Autodesk Inventor part; units mm, degrees
(part 3 of 3)
  point P86 (13.5104, 46.8405)
  point P87 (13.2211, 47.2236)
  point P88 (11.1615, 47.7468)
  point P89 (10.7263, 47.5553)
  point P90 (10.5426, 47.5964)
  point P91 (10.2298, 47.9606)
  point P92 (7.7191, 48.135)
  point P93 (7.5332, 48.1644)
  point P94 (7.1982, 48.5083)
  point P95 (5.0892, 48.7692)
  point P96 (4.6815, 48.5247)
  point P97 (4.4941, 48.5424)
  point P98 (4.1381, 48.8646)
  point P99 (2.0169, 48.9926)
  point P100 (1.6254, 48.7229)
  point P101 (1.4372, 48.7288)
  point P102 (1.0617, 49.028)
  point P103 (-1.0633, 49.0225)
  point P104 (-1.4372, 48.7288)
  point P105 (-1.6254, 48.7229)
  point P106 (-2.0189, 48.9979)
  point P107 (-2.8249, 50.9218)
  point P108 (-4.1394, 48.859)
  point P109 (-4.4941, 48.5424)
  point P110 (-4.6815, 48.5247)
  point P111 (-5.0915, 48.7745)
  point P112 (-6.0168, 50.6439)
  point P113 (-7.5332, 48.1644)
  point P114 (-7.7191, 48.135)
  point P115 (-8.144, 48.3585)
  point P116 (-9.1848, 50.1662)
  point P117 (-10.5426, 47.5964)
  point P118 (-10.7263, 47.5553)
  point P119 (-11.1644, 47.7517)
  point P120 (-12.3167, 49.4905)
  point P121 (-13.5104, 46.8405)
  point P122 (-13.6912, 46.788)
  point P123 (-14.1407, 46.9565)
  point P124 (-15.3999, 48.6194)
  point P125 (-16.1601, 46.2946)
  point P126 (-16.4249, 45.8997)
  point P127 (-16.602, 45.836)
  point P128 (-17.0612, 45.9759)
  point P129 (-18.4224, 47.5565)
  point P130 (-19.2745, 44.7778)
  point P131 (-19.4473, 44.7031)
  point P132 (-19.9144, 44.8139)
  point P133 (-21.3721, 46.3059)
  point P134 (-21.8349, 43.9042)
  point P135 (-22.0481, 43.4792)
  point P136 (-22.2159, 43.3938)
  point P137 (-24.2375, 44.8726)
  point P138 (-24.7347, 42.009)
  point P139 (-24.8967, 41.9132)
  point P140 (-25.3741, 41.9646)
  point P141 (-27.0072, 43.2622)
  point P142 (-27.1654, 40.8213)
  point P143 (-27.3237, 40.373)
  point P144 (-27.4794, 40.2672)
  point P145 (-27.959, 40.2885)
  point P146 (-29.6704, 41.481)
  point P147 (-29.6769, 39.0404)
  point P148 (-29.8048, 38.5777)
  point P149 (-29.9535, 38.4623)
  point P150 (-30.4336, 38.4535)
  point P151 (-32.0674, 37.0947)
  point P152 (-32.1683, 36.6301)
  point P153 (-32.3095, 36.5056)
  point P154 (-32.788, 36.4667)
  point P155 (-34.6354, 37.4352)
  point P156 (-34.4048, 34.5379)
  point P157 (-34.5379, 34.4048)
  point P158 (-35.0131, 34.3359)
  point P159 (-36.9176, 35.1866)
  point P160 (-36.5056, 32.3095)
  point P161 (-36.6301, 32.1683)
  point P162 (-37.1, 32.0697)
  point P163 (-39.0542, 32.7991)
  point P164 (-38.4623, 29.9535)
  point P165 (-38.5777, 29.8048)
  point P166 (-39.0404, 29.6769)
  point P167 (-41.0366, 30.2821)
  point P168 (-40.2851, 27.9545)
  point P169 (-40.2672, 27.4794)
  point P170 (-40.373, 27.3237)
  point P171 (-40.8268, 27.1669)
  point P172 (-42.857, 27.6457)
  point P173 (-41.9132, 24.8967)
  point P174 (-42.009, 24.7347)
  point P175 (-42.4521, 24.5498)
  point P176 (-43.471, 22.685)
  point P177 (-43.3938, 22.2159)
  point P178 (-43.4792, 22.0481)
  point P179 (-43.9098, 21.8358)
  point P180 (-45.984, 22.0563)
  point P181 (-44.7031, 19.4473)
  point P182 (-44.7778, 19.2745)
  point P183 (-45.1942, 19.0356)
  point P184 (-47.2782, 19.1254)
  point P185 (-45.836, 16.602)
  point P186 (-45.8997, 16.4249)
  point P187 (-46.3003, 16.1602)
  point P188 (-48.3858, 16.119)
  point P189 (-46.788, 13.6912)
  point P190 (-46.8405, 13.5104)
  point P191 (-47.2236, 13.2211)
  point P192 (-47.7468, 11.1615)
  point P193 (-47.5553, 10.7263)
  point P194 (-47.5964, 10.5426)
  point P195 (-47.9606, 10.2298)
  point P196 (-50.0245, 9.9276)
  point P197 (-48.135, 7.7191)
  point P198 (-48.1644, 7.5332)
  point P199 (-48.5083, 7.1982)
  constraints: 800 point on circle, 400 centre point, 600 other
extrude "Extrusion1" add sketch "Sketch1" along normal blind 7
sketch "Sketch10" plane through (0, 0, 7) normal (0, 0, 1) x (1, 0, 0)
  arc A0 (6.577, -1.5182) -> (6.6574, -1.1143) centre (0, 0) ccw
  arc A1 (7.0958, -0.7827) -> (6.6574, -1.1143) centre (7.0519, -1.1803) ccw
  line L0 (7.0958, -0.7827) -> (7.489, -0.8261)
  spline S0 degree 3 poles (7.489, -0.8261) (7.5332, -0.828) (7.6661, -0.828) (7.8888, -0.7776) knots 0 0 0 0 1 1 1 1
  line L1 (7.489, -0.8261) -> (7.5332, -0.828) construction
  line L2 (7.5332, -0.828) -> (7.6661, -0.828) construction
  line L3 (7.6661, -0.828) -> (7.8888, -0.7776) construction
  spline S1 degree 3 poles (7.8888, -0.7776) (8.1533, -0.7172) (8.5333, -0.5858) (8.996, -0.3043) knots 0 0 0 0 1 1 1 1
  line L4 (7.8888, -0.7776) -> (8.1533, -0.7172) construction
  line L5 (8.1533, -0.7172) -> (8.5333, -0.5858) construction
  line L6 (8.5333, -0.5858) -> (8.996, -0.3043) construction
  arc A2 (8.996, -0.3043) -> (8.996, 0.3043) centre (0, 0) ccw
  spline S2 degree 3 poles (8.996, 0.3043) (8.5333, 0.5858) (8.1533, 0.7172) (7.8888, 0.7776) knots 0 0 0 0 1 1 1 1
  line L7 (8.996, 0.3043) -> (8.5333, 0.5858) construction
  line L8 (8.5333, 0.5858) -> (8.1533, 0.7172) construction
  line L9 (8.1533, 0.7172) -> (7.8888, 0.7776) construction
  spline S3 degree 3 poles (7.8888, 0.7776) (7.6661, 0.828) (7.5332, 0.828) (7.489, 0.8261) knots 0 0 0 0 1 1 1 1
  line L10 (7.8888, 0.7776) -> (7.6661, 0.828) construction
  line L11 (7.6661, 0.828) -> (7.5332, 0.828) construction
  line L12 (7.5332, 0.828) -> (7.489, 0.8261) construction
  line L13 (7.489, 0.8261) -> (7.0958, 0.7827)
  arc A3 (6.6574, 1.1143) -> (7.0958, 0.7827) centre (7.0519, 1.1803) ccw
  arc A4 (6.6574, 1.1143) -> (6.577, 1.5182) centre (0, 0) ccw
  arc A5 (6.8552, 1.9923) -> (6.577, 1.5182) centre (6.9668, 1.6082) ccw
  line L14 (6.8552, 1.9923) -> (7.2351, 2.1027)
  spline S4 degree 3 poles (7.2351, 2.1027) (7.2766, 2.1178) (7.3994, 2.1687) (7.5858, 2.3005) knots 0 0 0 0 1 1 1 1
  line L15 (7.2351, 2.1027) -> (7.2766, 2.1178) construction
  line L16 (7.2766, 2.1178) -> (7.3994, 2.1687) construction
  line L17 (7.3994, 2.1687) -> (7.5858, 2.3005) construction
  spline S5 degree 3 poles (7.5858, 2.3005) (7.8072, 2.4576) (8.1079, 2.7244) (8.4277, 3.1615) knots 0 0 0 0 1 1 1 1
  line L18 (7.5858, 2.3005) -> (7.8072, 2.4576) construction
  line L19 (7.8072, 2.4576) -> (8.1079, 2.7244) construction
  line L20 (8.1079, 2.7244) -> (8.4277, 3.1615) construction
  arc A6 (8.4277, 3.1615) -> (8.1948, 3.7238) centre (0, 0) ccw
  spline S6 degree 3 poles (8.1948, 3.7238) (7.6596, 3.8067) (7.2583, 3.7827) (6.9907, 3.7373) knots 0 0 0 0 1 1 1 1
  line L21 (8.1948, 3.7238) -> (7.6596, 3.8067) construction
  line L22 (7.6596, 3.8067) -> (7.2583, 3.7827) construction
  line L23 (7.2583, 3.7827) -> (6.9907, 3.7373) construction
  spline S7 degree 3 poles (6.9907, 3.7373) (6.7657, 3.6986) (6.6429, 3.6478) (6.6028, 3.6291) knots 0 0 0 0 1 1 1 1
  line L24 (6.9907, 3.7373) -> (6.7657, 3.6986) construction
  line L25 (6.7657, 3.6986) -> (6.6429, 3.6478) construction
  line L26 (6.6429, 3.6478) -> (6.6028, 3.6291) construction
  line L27 (6.6028, 3.6291) -> (6.2561, 3.4386)
  arc A7 (5.7242, 3.5771) -> (6.2561, 3.4386) centre (6.0634, 3.7891) ccw
  arc A8 (5.7242, 3.5771) -> (5.4954, 3.9196) centre (0, 0) ccw
  arc A9 (5.5709, 4.464) -> (5.4954, 3.9196) centre (5.8211, 4.1518) ccw
  line L28 (5.5709, 4.464) -> (5.8797, 4.7114)
  spline S8 degree 3 poles (5.8797, 4.7114) (5.9123, 4.7413) (6.0062, 4.8353) (6.128, 5.0284) knots 0 0 0 0 1 1 1 1
  line L29 (5.8797, 4.7114) -> (5.9123, 4.7413) construction
  line L30 (5.9123, 4.7413) -> (6.0062, 4.8353) construction
  line L31 (6.0062, 4.8353) -> (6.128, 5.0284) construction
  spline S9 degree 3 poles (6.128, 5.0284) (6.2724, 5.2582) (6.4481, 5.6197) (6.5763, 6.146) knots 0 0 0 0 1 1 1 1
  line L32 (6.128, 5.0284) -> (6.2724, 5.2582) construction
  line L33 (6.2724, 5.2582) -> (6.4481, 5.6197) construction
  line L34 (6.4481, 5.6197) -> (6.5763, 6.146) construction
  arc A10 (6.5763, 6.146) -> (6.146, 6.5763) centre (0, 0) ccw
  spline S10 degree 3 poles (6.146, 6.5763) (5.6197, 6.4481) (5.2582, 6.2724) (5.0284, 6.128) knots 0 0 0 0 1 1 1 1
  line L35 (6.146, 6.5763) -> (5.6197, 6.4481) construction
  line L36 (5.6197, 6.4481) -> (5.2582, 6.2724) construction
  line L37 (5.2582, 6.2724) -> (5.0284, 6.128) construction
  spline S11 degree 3 poles (5.0284, 6.128) (4.8353, 6.0062) (4.7413, 5.9123) (4.7114, 5.8797) knots 0 0 0 0 1 1 1 1
  line L38 (5.0284, 6.128) -> (4.8353, 6.0062) construction
  line L39 (4.8353, 6.0062) -> (4.7413, 5.9123) construction
  line L40 (4.7413, 5.9123) -> (4.7114, 5.8797) construction
  line L41 (4.7114, 5.8797) -> (4.464, 5.5709)
  arc A11 (3.9196, 5.4954) -> (4.464, 5.5709) centre (4.1518, 5.8211) ccw
  arc A12 (3.9196, 5.4954) -> (3.5771, 5.7242) centre (0, 0) ccw
  arc A13 (3.4386, 6.2561) -> (3.5771, 5.7242) centre (3.7891, 6.0634) ccw
  line L42 (3.4386, 6.2561) -> (3.6291, 6.6028)
  spline S12 degree 3 poles (3.6291, 6.6028) (3.6478, 6.6429) (3.6986, 6.7657) (3.7373, 6.9907) knots 0 0 0 0 1 1 1 1
  line L43 (3.6291, 6.6028) -> (3.6478, 6.6429) construction
  line L44 (3.6478, 6.6429) -> (3.6986, 6.7657) construction
  line L45 (3.6986, 6.7657) -> (3.7373, 6.9907) construction
  spline S13 degree 3 poles (3.7373, 6.9907) (3.7827, 7.2583) (3.8067, 7.6596) (3.7238, 8.1948) knots 0 0 0 0 1 1 1 1
  line L46 (3.7373, 6.9907) -> (3.7827, 7.2583) construction
  line L47 (3.7827, 7.2583) -> (3.8067, 7.6596) construction
  line L48 (3.8067, 7.6596) -> (3.7238, 8.1948) construction
  arc A14 (3.7238, 8.1948) -> (3.1615, 8.4277) centre (0, 0) ccw
  spline S14 degree 3 poles (3.1615, 8.4277) (2.7244, 8.1079) (2.4576, 7.8072) (2.3005, 7.5858) knots 0 0 0 0 1 1 1 1
  line L49 (3.1615, 8.4277) -> (2.7244, 8.1079) construction
  line L50 (2.7244, 8.1079) -> (2.4576, 7.8072) construction
  line L51 (2.4576, 7.8072) -> (2.3005, 7.5858) construction
  spline S15 degree 3 poles (2.3005, 7.5858) (2.1687, 7.3994) (2.1178, 7.2766) (2.1027, 7.2351) knots 0 0 0 0 1 1 1 1
  line L52 (2.3005, 7.5858) -> (2.1687, 7.3994) construction
  line L53 (2.1687, 7.3994) -> (2.1178, 7.2766) construction
  line L54 (2.1178, 7.2766) -> (2.1027, 7.2351) construction
  line L55 (2.1027, 7.2351) -> (1.9923, 6.8552)
  arc A15 (1.5182, 6.577) -> (1.9923, 6.8552) centre (1.6082, 6.9668) ccw
  arc A16 (1.5182, 6.577) -> (1.1143, 6.6574) centre (0, 0) ccw
  arc A17 (0.7827, 7.0958) -> (1.1143, 6.6574) centre (1.1803, 7.0519) ccw
  line L56 (0.7827, 7.0958) -> (0.8261, 7.489)
  spline S16 degree 3 poles (0.8261, 7.489) (0.828, 7.5332) (0.828, 7.6661) (0.7776, 7.8888) knots 0 0 0 0 1 1 1 1
  line L57 (0.8261, 7.489) -> (0.828, 7.5332) construction
  line L58 (0.828, 7.5332) -> (0.828, 7.6661) construction
  line L59 (0.828, 7.6661) -> (0.7776, 7.8888) construction
  spline S17 degree 3 poles (0.7776, 7.8888) (0.7172, 8.1533) (0.5858, 8.5333) (0.3043, 8.996) knots 0 0 0 0 1 1 1 1
  line L60 (0.7776, 7.8888) -> (0.7172, 8.1533) construction
  line L61 (0.7172, 8.1533) -> (0.5858, 8.5333) construction
  line L62 (0.5858, 8.5333) -> (0.3043, 8.996) construction
  arc A18 (0.3043, 8.996) -> (-0.3043, 8.996) centre (0, 0) ccw
  spline S18 degree 3 poles (-0.3043, 8.996) (-0.5858, 8.5333) (-0.7172, 8.1533) (-0.7776, 7.8888) knots 0 0 0 0 1 1 1 1
  line L63 (-0.3043, 8.996) -> (-0.5858, 8.5333) construction
  line L64 (-0.5858, 8.5333) -> (-0.7172, 8.1533) construction
  line L65 (-0.7172, 8.1533) -> (-0.7776, 7.8888) construction
  spline S19 degree 3 poles (-0.7776, 7.8888) (-0.828, 7.6661) (-0.828, 7.5332) (-0.8261, 7.489) knots 0 0 0 0 1 1 1 1
  line L66 (-0.7776, 7.8888) -> (-0.828, 7.6661) construction
  line L67 (-0.828, 7.6661) -> (-0.828, 7.5332) construction
  line L68 (-0.828, 7.5332) -> (-0.8261, 7.489) construction
  line L69 (-0.8261, 7.489) -> (-0.7827, 7.0958)
  arc A19 (-1.1143, 6.6574) -> (-0.7827, 7.0958) centre (-1.1803, 7.0519) ccw
  arc A20 (-1.1143, 6.6574) -> (-1.5182, 6.577) centre (0, 0) ccw
  arc A21 (-1.9923, 6.8552) -> (-1.5182, 6.577) centre (-1.6082, 6.9668) ccw
  line L70 (-1.9923, 6.8552) -> (-2.1027, 7.2351)
  spline S20 degree 3 poles (-2.1027, 7.2351) (-2.1178, 7.2766) (-2.1687, 7.3994) (-2.3005, 7.5858) knots 0 0 0 0 1 1 1 1
  line L71 (-2.1027, 7.2351) -> (-2.1178, 7.2766) construction
  line L72 (-2.1178, 7.2766) -> (-2.1687, 7.3994) construction
  line L73 (-2.1687, 7.3994) -> (-2.3005, 7.5858) construction
  spline S21 degree 3 poles (-2.3005, 7.5858) (-2.4576, 7.8072) (-2.7244, 8.1079) (-3.1615, 8.4277) knots 0 0 0 0 1 1 1 1
  line L74 (-2.3005, 7.5858) -> (-2.4576, 7.8072) construction
  line L75 (-2.4576, 7.8072) -> (-2.7244, 8.1079) construction
  line L76 (-2.7244, 8.1079) -> (-3.1615, 8.4277) construction
  arc A22 (-3.1615, 8.4277) -> (-3.7238, 8.1948) centre (0, 0) ccw
  spline S22 degree 3 poles (-3.7238, 8.1948) (-3.8067, 7.6596) (-3.7827, 7.2583) (-3.7373, 6.9907) knots 0 0 0 0 1 1 1 1
  line L77 (-3.7238, 8.1948) -> (-3.8067, 7.6596) construction
  line L78 (-3.8067, 7.6596) -> (-3.7827, 7.2583) construction
  line L79 (-3.7827, 7.2583) -> (-3.7373, 6.9907) construction
  spline S23 degree 3 poles (-3.7373, 6.9907) (-3.6986, 6.7657) (-3.6478, 6.6429) (-3.6291, 6.6028) knots 0 0 0 0 1 1 1 1
  line L80 (-3.7373, 6.9907) -> (-3.6986, 6.7657) construction
  line L81 (-3.6986, 6.7657) -> (-3.6478, 6.6429) construction
  line L82 (-3.6478, 6.6429) -> (-3.6291, 6.6028) construction
  line L83 (-3.6291, 6.6028) -> (-3.4386, 6.2561)
  arc A23 (-3.5771, 5.7242) -> (-3.4386, 6.2561) centre (-3.7891, 6.0634) ccw
  arc A24 (-3.5771, 5.7242) -> (-3.9196, 5.4954) centre (0, 0) ccw
  arc A25 (-4.464, 5.5709) -> (-3.9196, 5.4954) centre (-4.1518, 5.8211) ccw
  line L84 (-4.464, 5.5709) -> (-4.7114, 5.8797)
  spline S24 degree 3 poles (-4.7114, 5.8797) (-4.7413, 5.9123) (-4.8353, 6.0062) (-5.0284, 6.128) knots 0 0 0 0 1 1 1 1
  line L85 (-4.7114, 5.8797) -> (-4.7413, 5.9123) construction
  line L86 (-4.7413, 5.9123) -> (-4.8353, 6.0062) construction
  line L87 (-4.8353, 6.0062) -> (-5.0284, 6.128) construction
  spline S25 degree 3 poles (-5.0284, 6.128) (-5.2582, 6.2724) (-5.6197, 6.4481) (-6.146, 6.5763) knots 0 0 0 0 1 1 1 1
  line L88 (-5.0284, 6.128) -> (-5.2582, 6.2724) construction
  line L89 (-5.2582, 6.2724) -> (-5.6197, 6.4481) construction
  line L90 (-5.6197, 6.4481) -> (-6.146, 6.5763) construction
  arc A26 (-6.146, 6.5763) -> (-6.5763, 6.146) centre (0, 0) ccw
  spline S26 degree 3 poles (-6.5763, 6.146) (-6.4481, 5.6197) (-6.2724, 5.2582) (-6.128, 5.0284) knots 0 0 0 0 1 1 1 1
  line L91 (-6.5763, 6.146) -> (-6.4481, 5.6197) construction
  line L92 (-6.4481, 5.6197) -> (-6.2724, 5.2582) construction
  line L93 (-6.2724, 5.2582) -> (-6.128, 5.0284) construction
  spline S27 degree 3 poles (-6.128, 5.0284) (-6.0062, 4.8353) (-5.9123, 4.7413) (-5.8797, 4.7114) knots 0 0 0 0 1 1 1 1
  line L94 (-6.128, 5.0284) -> (-6.0062, 4.8353) construction
  line L95 (-6.0062, 4.8353) -> (-5.9123, 4.7413) construction
  line L96 (-5.9123, 4.7413) -> (-5.8797, 4.7114) construction
  line L97 (-5.8797, 4.7114) -> (-5.5709, 4.464)
  arc A27 (-5.4954, 3.9196) -> (-5.5709, 4.464) centre (-5.8211, 4.1518) ccw
  arc A28 (-5.4954, 3.9196) -> (-5.7242, 3.5771) centre (0, 0) ccw
  arc A29 (-6.2561, 3.4386) -> (-5.7242, 3.5771) centre (-6.0634, 3.7891) ccw
  line L98 (-6.2561, 3.4386) -> (-6.6028, 3.6291)
  spline S28 degree 3 poles (-6.6028, 3.6291) (-6.6429, 3.6478) (-6.7657, 3.6986) (-6.9907, 3.7373) knots 0 0 0 0 1 1 1 1
  line L99 (-6.6028, 3.6291) -> (-6.6429, 3.6478) construction
  line L100 (-6.6429, 3.6478) -> (-6.7657, 3.6986) construction
  line L101 (-6.7657, 3.6986) -> (-6.9907, 3.7373) construction
  spline S29 degree 3 poles (-6.9907, 3.7373) (-7.2583, 3.7827) (-7.6596, 3.8067) (-8.1948, 3.7238) knots 0 0 0 0 1 1 1 1
  line L102 (-6.9907, 3.7373) -> (-7.2583, 3.7827) construction
  line L103 (-7.2583, 3.7827) -> (-7.6596, 3.8067) construction
  line L104 (-7.6596, 3.8067) -> (-8.1948, 3.7238) construction
  arc A30 (-8.1948, 3.7238) -> (-8.4277, 3.1615) centre (0, 0) ccw
  spline S30 degree 3 poles (-8.4277, 3.1615) (-8.1079, 2.7244) (-7.8072, 2.4576) (-7.5858, 2.3005) knots 0 0 0 0 1 1 1 1
  line L105 (-8.4277, 3.1615) -> (-8.1079, 2.7244) construction
  line L106 (-8.1079, 2.7244) -> (-7.8072, 2.4576) construction
  line L107 (-7.8072, 2.4576) -> (-7.5858, 2.3005) construction
  spline S31 degree 3 poles (-7.5858, 2.3005) (-7.3994, 2.1687) (-7.2766, 2.1178) (-7.2351, 2.1027) knots 0 0 0 0 1 1 1 1
  line L108 (-7.5858, 2.3005) -> (-7.3994, 2.1687) construction
  line L109 (-7.3994, 2.1687) -> (-7.2766, 2.1178) construction
  line L110 (-7.2766, 2.1178) -> (-7.2351, 2.1027) construction
  line L111 (-7.2351, 2.1027) -> (-6.8552, 1.9923)
  arc A31 (-6.577, 1.5182) -> (-6.8552, 1.9923) centre (-6.9668, 1.6082) ccw
  arc A32 (-6.577, 1.5182) -> (-6.6574, 1.1143) centre (0, 0) ccw
  arc A33 (-7.0958, 0.7827) -> (-6.6574, 1.1143) centre (-7.0519, 1.1803) ccw
  line L112 (-7.0958, 0.7827) -> (-7.489, 0.8261)
  spline S32 degree 3 poles (-7.489, 0.8261) (-7.5332, 0.828) (-7.6661, 0.828) (-7.8888, 0.7776) knots 0 0 0 0 1 1 1 1
  line L113 (-7.489, 0.8261) -> (-7.5332, 0.828) construction
  line L114 (-7.5332, 0.828) -> (-7.6661, 0.828) construction
  line L115 (-7.6661, 0.828) -> (-7.8888, 0.7776) construction
  spline S33 degree 3 poles (-7.8888, 0.7776) (-8.1533, 0.7172) (-8.5333, 0.5858) (-8.996, 0.3043) knots 0 0 0 0 1 1 1 1
  line L116 (-7.8888, 0.7776) -> (-8.1533, 0.7172) construction
  line L117 (-8.1533, 0.7172) -> (-8.5333, 0.5858) construction
  line L118 (-8.5333, 0.5858) -> (-8.996, 0.3043) construction
  arc A34 (-8.996, 0.3043) -> (-8.996, -0.3043) centre (0, 0) ccw
  spline S34 degree 3 poles (-8.996, -0.3043) (-8.5333, -0.5858) (-8.1533, -0.7172) (-7.8888, -0.7776) knots 0 0 0 0 1 1 1 1
  line L119 (-8.996, -0.3043) -> (-8.5333, -0.5858) construction
  line L120 (-8.5333, -0.5858) -> (-8.1533, -0.7172) construction
  line L121 (-8.1533, -0.7172) -> (-7.8888, -0.7776) construction
  spline S35 degree 3 poles (-7.8888, -0.7776) (-7.6661, -0.828) (-7.5332, -0.828) (-7.489, -0.8261) knots 0 0 0 0 1 1 1 1
  line L122 (-7.8888, -0.7776) -> (-7.6661, -0.828) construction
  line L123 (-7.6661, -0.828) -> (-7.5332, -0.828) construction
  line L124 (-7.5332, -0.828) -> (-7.489, -0.8261) construction
  line L125 (-7.489, -0.8261) -> (-7.0958, -0.7827)
  arc A35 (-6.6574, -1.1143) -> (-7.0958, -0.7827) centre (-7.0519, -1.1803) ccw
  arc A36 (-6.6574, -1.1143) -> (-6.577, -1.5182) centre (0, 0) ccw
  arc A37 (-6.8552, -1.9923) -> (-6.577, -1.5182) centre (-6.9668, -1.6082) ccw
  line L126 (-6.8552, -1.9923) -> (-7.2351, -2.1027)
  spline S36 degree 3 poles (-7.2351, -2.1027) (-7.2766, -2.1178) (-7.3994, -2.1687) (-7.5858, -2.3005) knots 0 0 0 0 1 1 1 1
  line L127 (-7.2351, -2.1027) -> (-7.2766, -2.1178) construction
  line L128 (-7.2766, -2.1178) -> (-7.3994, -2.1687) construction
  line L129 (-7.3994, -2.1687) -> (-7.5858, -2.3005) construction
  spline S37 degree 3 poles (-7.5858, -2.3005) (-7.8072, -2.4576) (-8.1079, -2.7244) (-8.4277, -3.1615) knots 0 0 0 0 1 1 1 1
  line L130 (-7.5858, -2.3005) -> (-7.8072, -2.4576) construction
  line L131 (-7.8072, -2.4576) -> (-8.1079, -2.7244) construction
  line L132 (-8.1079, -2.7244) -> (-8.4277, -3.1615) construction
  arc A38 (-8.4277, -3.1615) -> (-8.1948, -3.7238) centre (0, 0) ccw
  spline S38 degree 3 poles (-8.1948, -3.7238) (-7.6596, -3.8067) (-7.2583, -3.7827) (-6.9907, -3.7373) knots 0 0 0 0 1 1 1 1
  line L133 (-8.1948, -3.7238) -> (-7.6596, -3.8067) construction
  line L134 (-7.6596, -3.8067) -> (-7.2583, -3.7827) construction
  line L135 (-7.2583, -3.7827) -> (-6.9907, -3.7373) construction
  spline S39 degree 3 poles (-6.9907, -3.7373) (-6.7657, -3.6986) (-6.6429, -3.6478) (-6.6028, -3.6291) knots 0 0 0 0 1 1 1 1
  line L136 (-6.9907, -3.7373) -> (-6.7657, -3.6986) construction
  line L137 (-6.7657, -3.6986) -> (-6.6429, -3.6478) construction
  line L138 (-6.6429, -3.6478) -> (-6.6028, -3.6291) construction
  line L139 (-6.6028, -3.6291) -> (-6.2561, -3.4386)
  arc A39 (-5.7242, -3.5771) -> (-6.2561, -3.4386) centre (-6.0634, -3.7891) ccw
  arc A40 (-5.7242, -3.5771) -> (-5.4954, -3.9196) centre (0, 0) ccw
  arc A41 (-5.5709, -4.464) -> (-5.4954, -3.9196) centre (-5.8211, -4.1518) ccw
  line L140 (-5.5709, -4.464) -> (-5.8797, -4.7114)
  spline S40 degree 3 poles (-5.8797, -4.7114) (-5.9123, -4.7413) (-6.0062, -4.8353) (-6.128, -5.0284) knots 0 0 0 0 1 1 1 1
  line L141 (-5.8797, -4.7114) -> (-5.9123, -4.7413) construction
  line L142 (-5.9123, -4.7413) -> (-6.0062, -4.8353) construction
  line L143 (-6.0062, -4.8353) -> (-6.128, -5.0284) construction
  spline S41 degree 3 poles (-6.128, -5.0284) (-6.2724, -5.2582) (-6.4481, -5.6197) (-6.5763, -6.146) knots 0 0 0 0 1 1 1 1
  line L144 (-6.128, -5.0284) -> (-6.2724, -5.2582) construction
  line L145 (-6.2724, -5.2582) -> (-6.4481, -5.6197) construction
  line L146 (-6.4481, -5.6197) -> (-6.5763, -6.146) construction
  arc A42 (-6.5763, -6.146) -> (-6.146, -6.5763) centre (0, 0) ccw
  spline S42 degree 3 poles (-6.146, -6.5763) (-5.6197, -6.4481) (-5.2582, -6.2724) (-5.0284, -6.128) knots 0 0 0 0 1 1 1 1
  line L147 (-6.146, -6.5763) -> (-5.6197, -6.4481) construction
  line L148 (-5.6197, -6.4481) -> (-5.2582, -6.2724) construction
  line L149 (-5.2582, -6.2724) -> (-5.0284, -6.128) construction
  spline S43 degree 3 poles (-5.0284, -6.128) (-4.8353, -6.0062) (-4.7413, -5.9123) (-4.7114, -5.8797) knots 0 0 0 0 1 1 1 1
  line L150 (-5.0284, -6.128) -> (-4.8353, -6.0062) construction
  line L151 (-4.8353, -6.0062) -> (-4.7413, -5.9123) construction
  line L152 (-4.7413, -5.9123) -> (-4.7114, -5.8797) construction
  line L153 (-4.7114, -5.8797) -> (-4.464, -5.5709)
  arc A43 (-3.9196, -5.4954) -> (-4.464, -5.5709) centre (-4.1518, -5.8211) ccw
  arc A44 (-3.9196, -5.4954) -> (-3.5771, -5.7242) centre (0, 0) ccw
  arc A45 (-3.4386, -6.2561) -> (-3.5771, -5.7242) centre (-3.7891, -6.0634) ccw
  line L154 (-3.4386, -6.2561) -> (-3.6291, -6.6028)
  spline S44 degree 3 poles (-3.6291, -6.6028) (-3.6478, -6.6429) (-3.6986, -6.7657) (-3.7373, -6.9907) knots 0 0 0 0 1 1 1 1
  line L155 (-3.6291, -6.6028) -> (-3.6478, -6.6429) construction
  line L156 (-3.6478, -6.6429) -> (-3.6986, -6.7657) construction
  line L157 (-3.6986, -6.7657) -> (-3.7373, -6.9907) construction
  spline S45 degree 3 poles (-3.7373, -6.9907) (-3.7827, -7.2583) (-3.8067, -7.6596) (-3.7238, -8.1948) knots 0 0 0 0 1 1 1 1
  line L158 (-3.7373, -6.9907) -> (-3.7827, -7.2583) construction
  line L159 (-3.7827, -7.2583) -> (-3.8067, -7.6596) construction
  line L160 (-3.8067, -7.6596) -> (-3.7238, -8.1948) construction
  arc A46 (-3.7238, -8.1948) -> (-3.1615, -8.4277) centre (0, 0) ccw
  spline S46 degree 3 poles (-3.1615, -8.4277) (-2.7244, -8.1079) (-2.4576, -7.8072) (-2.3005, -7.5858) knots 0 0 0 0 1 1 1 1
  line L161 (-3.1615, -8.4277) -> (-2.7244, -8.1079) construction
  line L162 (-2.7244, -8.1079) -> (-2.4576, -7.8072) construction
  line L163 (-2.4576, -7.8072) -> (-2.3005, -7.5858) construction
  spline S47 degree 3 poles (-2.3005, -7.5858) (-2.1687, -7.3994) (-2.1178, -7.2766) (-2.1027, -7.2351) knots 0 0 0 0 1 1 1 1
  line L164 (-2.3005, -7.5858) -> (-2.1687, -7.3994) construction
  line L165 (-2.1687, -7.3994) -> (-2.1178, -7.2766) construction
  line L166 (-2.1178, -7.2766) -> (-2.1027, -7.2351) construction
  line L167 (-2.1027, -7.2351) -> (-1.9923, -6.8552)
  arc A47 (-1.5182, -6.577) -> (-1.9923, -6.8552) centre (-1.6082, -6.9668) ccw
  arc A48 (-1.5182, -6.577) -> (-1.1143, -6.6574) centre (0, 0) ccw
  arc A49 (-0.7827, -7.0958) -> (-1.1143, -6.6574) centre (-1.1803, -7.0519) ccw
  line L168 (-0.7827, -7.0958) -> (-0.8261, -7.489)
  spline S48 degree 3 poles (-0.8261, -7.489) (-0.828, -7.5332) (-0.828, -7.6661) (-0.7776, -7.8888) knots 0 0 0 0 1 1 1 1
  line L169 (-0.8261, -7.489) -> (-0.828, -7.5332) construction
  line L170 (-0.828, -7.5332) -> (-0.828, -7.6661) construction
  line L171 (-0.828, -7.6661) -> (-0.7776, -7.8888) construction
  spline S49 degree 3 poles (-0.7776, -7.8888) (-0.7172, -8.1533) (-0.5858, -8.5333) (-0.3043, -8.996) knots 0 0 0 0 1 1 1 1
  line L172 (-0.7776, -7.8888) -> (-0.7172, -8.1533) construction
  line L173 (-0.7172, -8.1533) -> (-0.5858, -8.5333) construction
  line L174 (-0.5858, -8.5333) -> (-0.3043, -8.996) construction
  arc A50 (-0.3043, -8.996) -> (0.3043, -8.996) centre (0, 0) ccw
  spline S50 degree 3 poles (0.3043, -8.996) (0.5858, -8.5333) (0.7172, -8.1533) (0.7776, -7.8888) knots 0 0 0 0 1 1 1 1
  line L175 (0.3043, -8.996) -> (0.5858, -8.5333) construction
  line L176 (0.5858, -8.5333) -> (0.7172, -8.1533) construction
  line L177 (0.7172, -8.1533) -> (0.7776, -7.8888) construction
  spline S51 degree 3 poles (0.7776, -7.8888) (0.828, -7.6661) (0.828, -7.5332) (0.8261, -7.489) knots 0 0 0 0 1 1 1 1
  line L178 (0.7776, -7.8888) -> (0.828, -7.6661) construction
  line L179 (0.828, -7.6661) -> (0.828, -7.5332) construction
  line L180 (0.828, -7.5332) -> (0.8261, -7.489) construction
  line L181 (0.8261, -7.489) -> (0.7827, -7.0958)
  arc A51 (1.1143, -6.6574) -> (0.7827, -7.0958) centre (1.1803, -7.0519) ccw
  arc A52 (1.1143, -6.6574) -> (1.5182, -6.577) centre (0, 0) ccw
  arc A53 (1.9923, -6.8552) -> (1.5182, -6.577) centre (1.6082, -6.9668) ccw
  line L182 (1.9923, -6.8552) -> (2.1027, -7.2351)
  spline S52 degree 3 poles (2.1027, -7.2351) (2.1178, -7.2766) (2.1687, -7.3994) (2.3005, -7.5858) knots 0 0 0 0 1 1 1 1
  line L183 (2.1027, -7.2351) -> (2.1178, -7.2766) construction
  line L184 (2.1178, -7.2766) -> (2.1687, -7.3994) construction
  line L185 (2.1687, -7.3994) -> (2.3005, -7.5858) construction
  spline S53 degree 3 poles (2.3005, -7.5858) (2.4576, -7.8072) (2.7244, -8.1079) (3.1615, -8.4277) knots 0 0 0 0 1 1 1 1
  line L186 (2.3005, -7.5858) -> (2.4576, -7.8072) construction
  line L187 (2.4576, -7.8072) -> (2.7244, -8.1079) construction
  line L188 (2.7244, -8.1079) -> (3.1615, -8.4277) construction
  arc A54 (3.1615, -8.4277) -> (3.7238, -8.1948) centre (0, 0) ccw
  spline S54 degree 3 poles (3.7238, -8.1948) (3.8067, -7.6596) (3.7827, -7.2583) (3.7373, -6.9907) knots 0 0 0 0 1 1 1 1
  line L189 (3.7238, -8.1948) -> (3.8067, -7.6596) construction
  line L190 (3.8067, -7.6596) -> (3.7827, -7.2583) construction
  line L191 (3.7827, -7.2583) -> (3.7373, -6.9907) construction
  spline S55 degree 3 poles (3.7373, -6.9907) (3.6986, -6.7657) (3.6478, -6.6429) (3.6291, -6.6028) knots 0 0 0 0 1 1 1 1
  line L192 (3.7373, -6.9907) -> (3.6986, -6.7657) construction
  line L193 (3.6986, -6.7657) -> (3.6478, -6.6429) construction
  line L194 (3.6478, -6.6429) -> (3.6291, -6.6028) construction
  line L195 (3.6291, -6.6028) -> (3.4386, -6.2561)
  arc A55 (3.5771, -5.7242) -> (3.4386, -6.2561) centre (3.7891, -6.0634) ccw
  arc A56 (3.5771, -5.7242) -> (3.9196, -5.4954) centre (0, 0) ccw
  arc A57 (4.464, -5.5709) -> (3.9196, -5.4954) centre (4.1518, -5.8211) ccw
  line L196 (4.464, -5.5709) -> (4.7114, -5.8797)
  spline S56 degree 3 poles (4.7114, -5.8797) (4.7413, -5.9123) (4.8353, -6.0062) (5.0284, -6.128) knots 0 0 0 0 1 1 1 1
  line L197 (4.7114, -5.8797) -> (4.7413, -5.9123) construction
  line L198 (4.7413, -5.9123) -> (4.8353, -6.0062) construction
  line L199 (4.8353, -6.0062) -> (5.0284, -6.128) construction
  spline S57 degree 3 poles (5.0284, -6.128) (5.2582, -6.2724) (5.6197, -6.4481) (6.146, -6.5763) knots 0 0 0 0 1 1 1 1
  line L200 (5.0284, -6.128) -> (5.2582, -6.2724) construction
  line L201 (5.2582, -6.2724) -> (5.6197, -6.4481) construction
  line L202 (5.6197, -6.4481) -> (6.146, -6.5763) construction
  arc A58 (6.146, -6.5763) -> (6.5763, -6.146) centre (0, 0) ccw
  spline S58 degree 3 poles (6.5763, -6.146) (6.4481, -5.6197) (6.2724, -5.2582) (6.128, -5.0284) knots 0 0 0 0 1 1 1 1
  line L203 (6.5763, -6.146) -> (6.4481, -5.6197) construction
  line L204 (6.4481, -5.6197) -> (6.2724, -5.2582) construction
  line L205 (6.2724, -5.2582) -> (6.128, -5.0284) construction
  spline S59 degree 3 poles (6.128, -5.0284) (6.0062, -4.8353) (5.9123, -4.7413) (5.8797, -4.7114) knots 0 0 0 0 1 1 1 1
  line L206 (6.128, -5.0284) -> (6.0062, -4.8353) construction
  line L207 (6.0062, -4.8353) -> (5.9123, -4.7413) construction
  line L208 (5.9123, -4.7413) -> (5.8797, -4.7114) construction
  line L209 (5.8797, -4.7114) -> (5.5709, -4.464)
  arc A59 (5.4954, -3.9196) -> (5.5709, -4.464) centre (5.8211, -4.1518) ccw
  arc A60 (5.4954, -3.9196) -> (5.7242, -3.5771) centre (0, 0) ccw
  arc A61 (6.2561, -3.4386) -> (5.7242, -3.5771) centre (6.0634, -3.7891) ccw
  line L210 (6.2561, -3.4386) -> (6.6028, -3.6291)
  spline S60 degree 3 poles (6.6028, -3.6291) (6.6429, -3.6478) (6.7657, -3.6986) (6.9907, -3.7373) knots 0 0 0 0 1 1 1 1
  line L211 (6.6028, -3.6291) -> (6.6429, -3.6478) construction
  line L212 (6.6429, -3.6478) -> (6.7657, -3.6986) construction
  line L213 (6.7657, -3.6986) -> (6.9907, -3.7373) construction
  spline S61 degree 3 poles (6.9907, -3.7373) (7.2583, -3.7827) (7.6596, -3.8067) (8.1948, -3.7238) knots 0 0 0 0 1 1 1 1
  line L214 (6.9907, -3.7373) -> (7.2583, -3.7827) construction
  line L215 (7.2583, -3.7827) -> (7.6596, -3.8067) construction
  line L216 (7.6596, -3.8067) -> (8.1948, -3.7238) construction
  arc A62 (8.1948, -3.7238) -> (8.4277, -3.1615) centre (0, 0) ccw
  spline S62 degree 3 poles (8.4277, -3.1615) (8.1079, -2.7244) (7.8072, -2.4576) (7.5858, -2.3005) knots 0 0 0 0 1 1 1 1
  line L217 (8.4277, -3.1615) -> (8.1079, -2.7244) construction
  line L218 (8.1079, -2.7244) -> (7.8072, -2.4576) construction
  line L219 (7.8072, -2.4576) -> (7.5858, -2.3005) construction
  spline S63 degree 3 poles (7.5858, -2.3005) (7.3994, -2.1687) (7.2766, -2.1178) (7.2351, -2.1027) knots 0 0 0 0 1 1 1 1
  line L220 (7.5858, -2.3005) -> (7.3994, -2.1687) construction
  line L221 (7.3994, -2.1687) -> (7.2766, -2.1178) construction
  line L222 (7.2766, -2.1178) -> (7.2351, -2.1027) construction
  line L223 (7.2351, -2.1027) -> (6.8552, -1.9923)
  arc A63 (6.577, -1.5182) -> (6.8552, -1.9923) centre (6.9668, -1.6082) ccw
  point P0 (6.2561, -3.4386)
  point P1 (6.6067, -3.6309)
  point P2 (6.9979, -3.7385)
  point P3 (8.1948, -3.7238)
  point P4 (7.5858, -2.3005)
  point P5 (7.2351, -2.1027)
  point P6 (6.8552, -1.9923)
  point P7 (6.577, -1.5182)
  point P8 (6.6574, -1.1143)
  point P9 (7.0958, -0.7827)
  point P10 (7.4933, -0.8263)
  point P11 (7.8959, -0.7759)
  point P12 (7.8888, 0.7776)
  point P13 (7.0958, 0.7827)
  point P14 (6.6574, 1.1143)
  point P15 (6.577, 1.5182)
  point P16 (6.8552, 1.9923)
  point P17 (7.2391, 2.1042)
  point P18 (7.5918, 2.3048)
  point P19 (6.9907, 3.7373)
  point P20 (6.2561, 3.4386)
  point P21 (5.7242, 3.5771)
  point P22 (5.4954, 3.9196)
  point P23 (5.5709, 4.464)
  point P24 (5.8828, 4.7143)
  point P25 (6.1319, 5.0346)
  point P26 (6.5763, 6.146)
  point P27 (5.0284, 6.128)
  point P28 (4.464, 5.5709)
  point P29 (3.9196, 5.4954)
  point P30 (3.5771, 5.7242)
  point P31 (3.4386, 6.2561)
  point P32 (3.6309, 6.6067)
  point P33 (3.7385, 6.9979)
  point P34 (3.7238, 8.1948)
  point P35 (2.3005, 7.5858)
  point P36 (2.1027, 7.2351)
  point P37 (1.9923, 6.8552)
  point P38 (1.5182, 6.577)
  point P39 (1.1143, 6.6574)
  point P40 (0.7827, 7.0958)
  point P41 (0.8263, 7.4933)
  point P42 (0.7759, 7.8959)
  point P43 (-0.7776, 7.8888)
  point P44 (-0.7827, 7.0958)
  point P45 (-1.1143, 6.6574)
  point P46 (-1.5182, 6.577)
  point P47 (-1.9923, 6.8552)
  point P48 (-2.1042, 7.2391)
  point P49 (-2.3048, 7.5918)
  point P50 (-3.1615, 8.4277)
  point P51 (-3.7373, 6.9907)
  point P52 (-3.4386, 6.2561)
  point P53 (-3.5771, 5.7242)
  point P54 (-3.9196, 5.4954)
  point P55 (-4.464, 5.5709)
  point P56 (-4.7143, 5.8828)
  point P57 (-5.0346, 6.1319)
  point P58 (-6.128, 5.0284)
  point P59 (-5.5709, 4.464)
  point P60 (-5.4954, 3.9196)
  point P61 (-5.7242, 3.5771)
  point P62 (-6.2561, 3.4386)
  point P63 (-6.6067, 3.6309)
  point P64 (-6.9979, 3.7385)
  point P65 (-8.1948, 3.7238)
  point P66 (-7.5858, 2.3005)
  point P67 (-7.2351, 2.1027)
  point P68 (-6.8552, 1.9923)
  point P69 (-6.577, 1.5182)
  point P70 (-6.6574, 1.1143)
  point P71 (-7.0958, 0.7827)
  point P72 (-7.4933, 0.8263)
  point P73 (-7.8959, 0.7759)
  point P74 (-7.8888, -0.7776)
  point P75 (-7.0958, -0.7827)
  point P76 (-6.6574, -1.1143)
  point P77 (-6.577, -1.5182)
  point P78 (-6.8552, -1.9923)
  point P79 (-7.2391, -2.1042)
  point P80 (-7.5918, -2.3048)
  point P81 (-6.9907, -3.7373)
  point P82 (-6.2561, -3.4386)
  point P83 (-5.7242, -3.5771)
  point P84 (-5.4954, -3.9196)
  point P85 (-5.5709, -4.464)
  point P86 (-5.8828, -4.7143)
  point P87 (-6.1319, -5.0346)
  point P88 (-6.5763, -6.146)
  point P89 (-5.0284, -6.128)
  point P90 (-4.464, -5.5709)
  point P91 (-3.9196, -5.4954)
  point P92 (-3.5771, -5.7242)
  point P93 (-3.4386, -6.2561)
  point P94 (-3.6309, -6.6067)
  point P95 (-3.7385, -6.9979)
  point P96 (-3.7238, -8.1948)
  point P97 (-2.3005, -7.5858)
  point P98 (-2.1027, -7.2351)
  point P99 (-1.9923, -6.8552)
  point P100 (-1.5182, -6.577)
  point P101 (-1.1143, -6.6574)
  point P102 (-0.7827, -7.0958)
  point P103 (-0.8263, -7.4933)
  point P104 (-0.7759, -7.8959)
  point P105 (0.7776, -7.8888)
  point P106 (0.7827, -7.0958)
  point P107 (1.1143, -6.6574)
  point P108 (1.5182, -6.577)
  point P109 (1.9923, -6.8552)
  point P110 (2.1042, -7.2391)
  point P111 (2.3048, -7.5918)
  point P112 (3.7373, -6.9907)
  point P113 (3.4386, -6.2561)
  point P114 (3.5771, -5.7242)
  point P115 (3.9196, -5.4954)
  point P116 (4.464, -5.5709)
  point P117 (4.7143, -5.8828)
  point P118 (5.0346, -6.1319)
  point P119 (6.128, -5.0284)
  point P120 (5.8828, -4.7143)
  point P121 (5.5709, -4.464)
  point P122 (5.4954, -3.9196)
  point P123 (5.7242, -3.5771)
  constraints: 128 point on circle, 64 centre point, 64 end point, 192 other
extrude "Extrusion10" add sketch "Sketch10" along normal blind 8
sketch "Sketch11" plane through (0, 0, 15) normal (0, 0, 1) x (1, 0, 0)
  circle A0 centre (0, 0) radius 4
  dimension "d24" = 8
  constraints: 1 centre point, 1 coincident
  measures "d24" diameter of A0
extrude "Extrusion11" cut sketch "Sketch11" against normal blind 20
body "Solid1"
